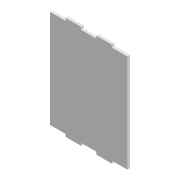
# Autodesk Inventor part: Top 1
Saved by Autodesk Inventor 2022 (Build 260153000, 153)
## iProperties
Created: 2022-06-06
Part Number: Top 1
Material: Generic
Document SubType Name: Modeling
Designer: ADMIN
Density: 1 g/cm^3
Appearance: Default
Author: ADMIN
Autodesk Inventor part; units mm, degrees
ref_plane "YZ Plane" through (0, 0, 0) normal (1, 0, 0) x (0, 1, 0)
ref_plane "XZ Plane" through (0, 0, 0) normal (0, 1, 0) x (-1, 0, 0)
ref_plane "XY Plane" through (0, 0, 0) normal (0, 0, 1) x (1, 0, 0)
sketch "Sketch1" plane through (0, 0, 0) normal (0, 0, 1) x (1, 0, 0)
  line L0 (0, 0) -> (150, 0) projected
  line L1 (150, 0) -> (150, 200) projected
  line L2 (0, 200) -> (150, 200) projected
  line L3 (0, 0) -> (0, 200) projected
  line L4 (30, 205) -> (60, 205) projected
  line L5 (30, 205) -> (30, 200) projected
  line L6 (60, 200) -> (30, 200) projected
  line L7 (60, 205) -> (60, 200) projected
  line L8 (90, 205) -> (120, 205) projected
  line L9 (90, 205) -> (90, 200) projected
  line L10 (120, 200) -> (90, 200) projected
  line L11 (120, 205) -> (120, 200) projected
  line L12 (60, 200) -> (30, 200)
  line L13 (30, 200) -> (30, 195)
  line L14 (30, 195) -> (60, 195)
  line L15 (60, 195) -> (60, 200)
  line L16 (120, 200) -> (90, 200)
  line L17 (90, 200) -> (90, 195)
  line L18 (90, 195) -> (120, 195)
  line L19 (120, 195) -> (120, 200)
  line L20 (0, 195) -> (150, 195)
  line L21 (150, 100) -> (0, 100)
  line L22 (60, 0) -> (30, 0)
  line L23 (120, 0) -> (90, 0)
  line L24 (30, 0) -> (30, 5)
  line L25 (60, 5) -> (60, 0)
  line L26 (90, 0) -> (90, 5)
  line L27 (120, 5) -> (120, 0)
  line L28 (0, 5) -> (150, 5)
  dimension "d0" = 30
  dimension "d1" = 5
  dimension "d2" = 30
  dimension "d3" = 5
  constraints: 34 end point, 12 symmetric about line, 4 parallel, 3 perpendicular, 2 horizontal, 2 midpoint, 2 point on line
  measures "d0" distance of L14.end L13.end
  measures "d1" distance of L13.end L12.end
  measures "d2" distance of L18.end L17.end
  measures "d3" distance of L17.end L16.end
extrude "Extrusion1" add sketch "Sketch1" along normal blind 5 contours L24 L28 L25 L0 | L3 L21 L1 L28 | L3 L20 L14 L18 L1 L21 | L26 L28 L27 L0 | L13 L2 L15 L14 | L18 L17 L2 L19
body "Solid1"
